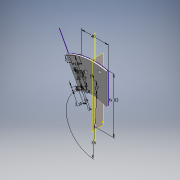
# Autodesk Inventor part: end_stop_40mm_v2
Saved by Autodesk Inventor 2016 (Build 200138000, 138)
## iProperties
Created: 2018-04-16
Part Number: end_stop_40mm_v2
Material: Generic
Document SubType Name: Modeling
Designer: mbouhier
Density: 1 g/cm^3
Appearance: Default
Author: mbouhier
Autodesk Inventor part; units mm, degrees
ref_plane "XZ Plane" through (0, 0, 0) normal (0, 1, 0) x (-1, 0, 0)
ref_plane "XY Plane" through (0, 0, 0) normal (0, 0, 1) x (1, 0, 0)
sketch "Sketch1" plane through (0, 0, 0) normal (0, 1, 0) x (-1, 0, 0)
  arc A0 (20, 38.0657) -> (0, 43) centre (0, 0) ccw
  line L0 (-20, 83) -> (20, 83)
  line L1 (20, 83) -> (20, 38.0657)
  line L2 (-20, 38.0657) -> (-20, 83)
  line L3 (-20, 83) -> (20, 38.0657) construction
  line L4 (20, 83) -> (-20, 38.0657) construction
  line L5 (24.2906, 35.4819) -> (26.151, 39.0229)
  line L6 (0, -20.3907) -> (0, 122.3444) projected
  line L7 (20, 38.0657) -> (53.5672, 101.9537)
  line L8 (5.836, 45.5076) -> (20, 38.0657)
  line L9 (20, 38.0657) -> (38.3721, 73.0331)
  line L10 (38.3721, 73.0331) -> (24.2081, 80.475)
  line L11 (20, 38.0657) -> (14.6885, 40.8564)
  line L12 (14.6885, 40.8564) -> (26.7815, 63.8729)
  line L13 (26.7815, 63.8729) -> (32.093, 61.0822)
  line L14 (32.093, 61.0822) -> (20, 38.0657)
  arc A1 (39.7096, 75.5788) -> (-20, 83) centre (0, 0) ccw
  line L15 (26.151, 39.0229) -> (21.7248, 41.3485)
  line L16 (1.8343, 42.9609) -> (1.8343, 59.9609)
  line L17 (1.8343, 59.9609) -> (5.8341, 60)
  line L18 (10.6171, 42.9956) -> (10, 41.821)
  line L19 (5.8341, 60) -> (13.4504, 60)
  line L20 (13.4504, 60) -> (5.836, 45.5076)
  line L21 (15.4217, 42.2519) -> (14.4928, 40.484)
  arc A2 (24.2906, 35.4819) -> (-20, 38.0657) centre (0, 0) ccw
  circle A3 centre (27.8094, 59.3792) radius 1.9
  circle A4 centre (18.9722, 42.5595) radius 1.9
  line L22 (34.6512, 65.9511) -> (20.4872, 73.393)
  line L23 (10.2623, 43.182) -> (22.3553, 66.1985)
  line L24 (22.3553, 66.1985) -> (17.929, 68.5241)
  line L25 (24.2081, 80.475) -> (20, 72.4657)
  line L26 (17.929, 68.5241) -> (5.836, 45.5076)
  point P0 (0, 60.5329)
  point P1 (0, 60.5329)
  point P2 (24.9134, 71.0674)
  dimension "d0" = 86
  dimension "d5" = 40
  dimension "d17" = 16
  dimension "d18" = 39.5
  dimension "d19" = 6
  dimension "d20" = 26
  dimension "d21" = 3
  dimension "d22" = 3
  dimension "d23" = 19
  dimension "d24" = 3.5
  dimension "d25" = 83
  dimension "d27" = 5
  dimension "d28" = 4
  dimension "d29" = 17
  dimension "d36" = 4
  dimension "d37" = 3.8
  dimension "d38" = 3.8
  dimension "d41" = 8
  constraints: 52 end point, 12 point on line, 11 point on circle, 10 perpendicular, 9 parallel, 5 centre point, 5 coincident, 3 midpoint, 2 collinear, 2 horizontal, 1 tangent
  measures "d0" diameter of A0
  measures "d5" distance of L0.start L0.end
  measures "d17" distance of L10.end L9.end
  measures "d18" distance of L1.end L9.end
  measures "d19" distance of L12.end L13.end
  measures "d20" distance of L11.end L12.end
  measures "d21" distance from line of point (18.972, 42.559) L14
  measures "d22" distance from line of point (27.809, 59.379) L14
  measures "d23" distance of point (27.809, 59.379) point (18.972, 42.559)
  measures "d24" distance from line of L8 point (18.972, 42.559)
  measures "d25" distance from line of L0 point (0, 0)
  measures "d27" distance of L5.end L15.end
  measures "d28" distance of L16.end L17.end
  measures "d29" distance of L16.start L16.end
  measures "d36" distance of L5.start L5.end
  measures "d37" diameter of A3
  measures "d38" diameter of A4
  measures "d41" distance from line of L22.start L10
extrude "Extrusion1" add sketch "Sketch1" against normal blind 3 contours L8 L12 L1 A4 | L1 A4 L12 L13 L7 | A0 L21 L8 | L7 L15 L5 A2 | A0 L18 L8 L21 | A4 L1 | L1 A4 | L8 L23 L1 L12 | A0 L16 L17 L19 L20 L8 L18 | L13 L12 L1 L23 L24 L25 L22 L7 | A0 L6 L0 L1 L24 L26 L19 L17 L16 | L22 L25 L10 L7 | L8 L20 L26 L24 L1 L23 | A2 L2 L0 L6 | L1 L24 L23 | L10 L25 L1 A1 L7 | L6 A1 L0 | L0 A1 L6 | A3
extrude "Extrusion2" add sketch "Sketch1" along normal blind 12 contours L7 L15 L5 A2 | A0 L16 L17 L19 L20 L8 L18
extrude "Extrusion3" add sketch "Sketch1" along normal blind 4 contours L8 L12 L1 A4 | L1 A4 L12 L13 L7 | A0 L21 L8 | A4 L1 | L1 A4 | A0 L16 L17 L19 L20 L8 L18 | L22 L25 L10 L7 | L8 L20 L26 L24 L1 L23 | L1 L24 L23 | A3
extrude "Extrusion4" cut sketch "Sketch1" along normal through all both and the other way through all contours A4 L1 | L1 A4 | A3
sketch "Sketch3" plane through (0, 0, 0) normal (0, 1, 0) x (1, 0, 0)
  line L0 (20, -83) -> (20, -38.0657) projected
  line L1 (20, -83) -> (-20, -83) projected
  arc A0 (-1.8343, -42.9609) -> (20, -38.0657) centre (0, 0) ccw projected
  line L2 (-20, -83) -> (-20, -38.0657) projected
  line L3 (-13.4504, -60) -> (-5.8341, -60) projected
  point P0 (10, -78)
  point P1 (10, -58)
  point P2 (10, -41.821)
  point P3 (-10, -49.821)
  point P4 (-10, -68)
  dimension "d51" = 10
  dimension "d52" = 10
  dimension "d53" = 5
  dimension "d56" = 10
  dimension "d70" = 25
  dimension "d73" = 20
  dimension "d74" = 10
  constraints: 1 point on circle
  measures "d51" distance from line of point (10, -78) L0
  measures "d52" distance from line of point (10, -58) L0
  measures "d53" distance from line of point (10, -78) L1
  measures "d56" distance from line of point (-10, -68) L2
  measures "d70" distance from line of point (10, -58) L1
  measures "d73" distance of point (10, -58) point (10, -78)
  measures "d74" vertical distance of point (-10, -68) point (10, -78)
hole "Hole1" at (-10, 0, 68) at (10, 0, 78) direction (0, -1, 0) diameter 4.5 end through all
sketch "Sketch5" plane through (0, 12, 0) normal (0, 1, 0) x (1, 0, 0)
  point P0 (0, 0)
sketch "Sketch6" plane through (0, 12, 0) normal (0, 1, 0) x (1, 0, 0)
  line L0 (-5.4309, -45.3816) -> (-20.126, -37.6606)
  line L1 (-20.126, -37.6606) -> (-30.0576, -56.5632)
  line L2 (-30.0576, -56.5632) -> (-15.3625, -64.2842)
  line L3 (-15.3625, -64.2842) -> (-5.4309, -45.3816)
  line L4 (-10.6171, -42.9956) -> (-5.836, -45.5076) projected
  line L5 (-5.836, -45.5076) -> (-13.4504, -60) projected
  line L6 (-21.7248, -41.3485) -> (-20, -38.0657) projected
  point P0 (0, 0)
  dimension "d65" = 0.3
  dimension "d66" = 0.3
  dimension "d69" = 0.3
  constraints: 8 end point, 2 parallel, 1 perpendicular
  measures "d65" distance between parallel lines of L0 L4
  measures "d66" distance between parallel lines of L3 L5
  measures "d69" distance between parallel lines of L6 L1
extrude "ajustement" cut sketch "Sketch6" against normal up to surface (8 mm away)
equation "\"d74\" = 0.5 * d73"
body "Solid1"
